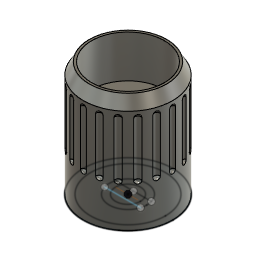
NXI Outer Knob v2 (Autodesk Fusion 360 design; units mm, degrees)
Autodesk Fusion 360 part; units mm, degrees
sketch "Sketch1" plane through (0, 0, 0) normal (0, 1, 0) x (1, 0, 0)
  circle A0 centre (0, 0) radius 7.4
  circle A1 centre (0, 0) radius 6.2
  circle A2 centre (0, 0) radius 3.1
  circle A3 centre (0, 0) radius 2.05
  line L0 (0, 0) -> (0, 0.9) construction
  line L1 (2.971, 0.9) -> (-2.9665, 0.9)
  line L2 (-2.05, 0) -> (2.05, 0) construction
  line L3 (2.971, -0.9) -> (-2.9665, -0.9)
  dimension "d1" = 14.8
  dimension "d2" = 12.4
  dimension "d3" = 6.2
  dimension "d4" = 4.1
  dimension "d18" = 0.9
  constraint coincident A0.centre A1.centre
  constraint concentric A1 A2
  constraint vertical L0
  constraint perpendicular L0 L1
  constraint coincident A3 L2.start
  constraint coincident A3 L2.end
  constraint perpendicular L0 L2
  constraint coincident A2 L1.end
  constraint symmetric L1.start L2 L3.start
  constraint symmetric L1.end L2 L3.end
  measures "d1" diameter of A0
  measures "d2" diameter of A1
  measures "d3" diameter of A2
  measures "d4" diameter of A3
  measures "d18" distance of A0.centre L1
extrude "Extrude1" add sketch "Sketch1" along normal blind 19 contours A0 | A1 | A2 A3 L1 L3 | A2 A3 L1 | A2 A3 L3 | A2 A3 L1 L3 | A3 L1 L3 | A3 L1 | A3 L3 makes body 1
extrude "Extrude2" cut sketch "Sketch1" along normal blind 4.7 contours A1 | A2 A3 L1 L3 | A2 A3 L1 | A2 A3 L3 | A2 A3 L1 L3 | A3 L1 L3 | A3 L1 | A3 L3 bodies 1
extrude "Extrude3" cut sketch "Sketch1" along normal up to surface (19 mm away) contours A2 A3 L1 | A2 A3 L3 | A3 L1 L3 | A3 L1 | A3 L3 bodies 1
sketch "Sketch2" plane through (0, 19, 0) normal (0, 1, 0) x (-1, 0, 0)
  arc A0 (1.8419, -0.9) -> (1.8419, 0.9) centre (0, 0) ccw
  line L0 (1.8419, -0.9) -> (2.9665, -0.9)
  circle A1 centre (0, 0) radius 7.4
  circle A2 centre (0, 0) radius 6.025
  line L1 (-1.8419, 0.9) -> (-2.9665, 0.9)
  arc A3 (2.9665, 0.9) -> (-2.9665, 0.9) centre (0, 0) ccw
  line L2 (2.9665, 0.9) -> (1.8419, 0.9)
  arc A4 (-2.9665, -0.9) -> (2.9665, -0.9) centre (0, 0) ccw
  line L3 (-2.9665, -0.9) -> (-1.8419, -0.9)
  arc A5 (-1.8419, 0.9) -> (-1.8419, -0.9) centre (0, 0) ccw
  dimension "d12" = 12.05
  constraint concentric A0 A2
  measures "d12" diameter of A2
extrude "Extrude4" cut sketch "Sketch2" against normal blind 7 contours A2 bodies 1
extrude "Extrude5" cut sketch "Sketch1" along normal blind 2.7 from surface at 4.7 contours A2 A3 L1 L3 | A2 A3 L1 | A2 A3 L3 | A2 A3 L1 L3 | A3 L1 bodies 1
chamfer "Chamfer1" distance 1 angle 62 1 edges at (-6.8992, 19, 2.676) measured on face at (6.8917, 19, 0.667) on bodies 1
sketch "Sketch3" plane through (0, 0, 0) normal (0, 0, 1) x (1, 0, 0)
  line L0 (10, 20) -> (10, 11)
  arc A0 (9.5, 10.5) -> (10, 11) centre (9.5, 11) ccw
  arc A1 (10, 20) -> (9.5, 20.5) centre (9.5, 20) ccw
  line L1 (9.5, 20.5) -> (9.5, 10.5)
  dimension "d23" = 9
  constraint vertical L0
  constraint tangent L0 A0
  constraint tangent L0 A1
  measures "d23" distance of L0.start L0.end
revolve "Revolve1" add sketch "Sketch3" angle 360 about axis through (9.5, 20.5, 0) along (0, -1, 0) separate body makes body 2
move_body "Move1" bodies 2 to x (1, 0, 0) y (0, 1, 0) z (0, 0, 1) at (-2, -3.9, 0)
pattern_circular "C-Pattern1" count 20 over 360 about axis through (0, 0, 0) along (0, 1, 0) of bodies 2 makes body 3 at (7.6002, 13.1, -2.4956) makes body 4 at (6.457, 13.1, -4.7221) makes body 5 at (4.6818, 13.1, -6.4863) makes body 6 at (2.4482, 13.1, -7.6156) makes body 7 at (-0.0249, 13.1, -7.9994) makes body 8 at (-2.4956, 13.1, -7.6002) makes body 9 at (-4.7221, 13.1, -6.457) makes body 10 at (-6.4863, 13.1, -4.6818) makes body 11 at (-7.6156, 13.1, -2.4482) makes body 12 at (-7.9994, 13.1, 0.0249) makes body 13 at (-7.6002, 13.1, 2.4956) makes body 14 at (-6.457, 13.1, 4.7221) makes body 15 at (-4.6818, 13.1, 6.4863) makes body 16 at (-2.4482, 13.1, 7.6156) makes body 17 at (0.0249, 13.1, 7.9994) makes body 18 at (2.4956, 13.1, 7.6002) makes body 19 at (4.7221, 13.1, 6.457) makes body 20 at (6.4863, 13.1, 4.6818) makes body 21 at (7.6156, 13.1, 2.4482)
combine "Combine1" operation cut target body 1 tool bodies 2 5 4 3 15 11 8 9 12 13 14 6 10 7 16 21 19 17 18 20
equation "d13 = ( -7 / 1 ) * 1 mm"
